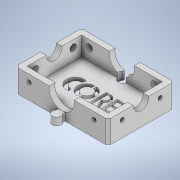
# Autodesk Inventor part: Rack holder aluminium
Saved by Autodesk Inventor 2021 (Build 250183000, 183)
## iProperties
Created: 2021-05-21
Part Number: Rack holder aluminium
Material: Generic
Document SubType Name: Modeling
Designer: Olivi
Density: 1 g/cm^3
Appearance: Default
Author: Olivi
Autodesk Inventor part; units mm, degrees
ref_plane "YZ Plane" through (0, 0, 0) normal (1, 0, 0) x (0, 1, 0)
ref_plane "XZ Plane" through (0, 0, 0) normal (0, 1, 0) x (-1, 0, 0)
ref_plane "XY Plane" through (0, 0, 0) normal (0, 0, 1) x (1, 0, 0)
sketch "Sketch1" plane through (0, 0, 0) normal (0, 1, 0) x (-1, 0, 0)
  line L0 (0, 0) -> (0, -86)
  line L1 (0, -86) -> (128.3, -86)
  line L2 (128.3, -86) -> (128.3, 0)
  line L3 (128.3, 0) -> (0, 0)
  dimension "d0" = 86
  dimension "d1" = 128.3
  constraints: 8 end point, 3 perpendicular, 1 vertical
  measures "d0" distance of L0.start L0.end
  measures "d1" distance of L0.end L1.end
extrude "Extrusion2" add sketch "Sketch1" along normal blind 6
sketch "Sketch3" plane through (0, 6, 0) normal (0, 1, 0) x (1, 0, 0)
  point P0 (0, 0)
sketch "Sketch4" plane through (0, 6, 0) normal (0, 1, 0) x (1, 0, 0)
  arc A0 (-91.2531, 56.696) -> (-91.5743, 29.7143) centre (-95.2962, 43.2514) ccw
  arc A1 (-93.1804, 51.2354) -> (-93.1804, 34.2112) centre (-94.0166, 42.7233) ccw
  line L0 (-93.1804, 51.2354) -> (-91.2531, 56.696)
  line L1 (-93.1804, 34.2112) -> (-91.5743, 29.7143)
  arc A2 (-78.0632, 52.0407) -> (-78.3199, 34.448) centre (-76.5372, 43.2202) ccw
  arc A3 (-74.7545, 34.448) -> (-75.0113, 52.0407) centre (-76.5372, 43.2202) ccw
  arc A4 (-75.0113, 29.7143) -> (-75.0113, 56.696) centre (-76.1328, 43.2051) ccw
  line L2 (-75.0113, 56.696) -> (-75.0113, 52.0407)
  line L3 (-74.7545, 34.448) -> (-75.0113, 29.7143)
  line L4 (-78.3199, 34.448) -> (-78.3199, 29.4603)
  line L5 (-78.0632, 56.6961) -> (-78.0632, 52.0407)
  arc A5 (-78.0632, 56.6961) -> (-78.3199, 29.4603) centre (-77.9302, 43.0757) ccw
  line L6 (-59.5494, 56.6961) -> (-59.5494, 29.4603)
  line L7 (-59.5494, 29.4603) -> (-55.5494, 29.4603)
  line L8 (-55.5494, 29.4603) -> (-55.5494, 56.6961)
  line L9 (-55.5494, 56.6961) -> (-59.5494, 56.6961)
  line L10 (-47.4135, 29.4603) -> (-53.7861, 43.0782)
  arc A6 (-53.7861, 43.0782) -> (-53.7861, 54.3684) centre (-53.0876, 48.7233) ccw
  line L11 (-47.4135, 29.4603) -> (-43.9803, 31.0669)
  line L12 (-43.9803, 31.0669) -> (-48.5954, 40.9288)
  arc A7 (-48.5954, 40.9288) -> (-53.7861, 56.6961) centre (-52.5494, 48.3652) ccw
  line L13 (-53.7861, 56.6961) -> (-53.7861, 54.3684)
  line L14 (-41.5494, 56.0046) -> (-41.5494, 29.4603)
  line L15 (-41.5494, 29.4603) -> (-27.5494, 29.4603)
  line L16 (-27.5494, 29.4603) -> (-27.5494, 33.1666)
  line L17 (-27.5494, 33.1666) -> (-37.5494, 33.1666)
  line L18 (-37.5494, 33.1666) -> (-37.5494, 41.4179)
  line L19 (-37.5494, 41.4179) -> (-29.2175, 41.4179)
  line L20 (-29.2175, 41.4179) -> (-29.2175, 44.4179)
  line L21 (-29.2175, 44.4179) -> (-37.5494, 44.4179)
  line L22 (-37.5494, 44.4179) -> (-37.5494, 52.4179)
  line L23 (-37.5494, 52.4179) -> (-27.5494, 52.4179)
  line L24 (-27.5494, 52.4179) -> (-27.5494, 56.0046)
  line L25 (-27.5494, 56.0046) -> (-41.5494, 56.0046)
  line L26 (-128.3, 86) -> (-128.3, 0) projected
  line L27 (0, 86) -> (-128.3, 86) projected
  point P0 (0, 0)
  constraints: 52 end point, 19 point on circle, 13 perpendicular, 8 centre point, 6 vertical, 5 point on line, 1 concentric
extrude "Extrusion3" cut sketch "Sketch4" against normal through all
sketch "Sketch26" plane through (0, 6, 0) normal (0, 1, 0) x (1, 0, 0)
  point P0 (0, 0)
sketch "Sketch27" plane through (0, 6, 0) normal (0, 1, 0) x (1, 0, 0)
  line L0 (-1.7618, -2.4025) -> (1.922, -2.4025)
  point P0 (0, 0)
  constraints: 2 end point, 1 horizontal
sketch "Sketch28" plane through (0, 6, 0) normal (0, 1, 0) x (1, 0, 0)
  point P0 (0, 0)
sketch "Sketch29" plane through (0, 6, 0) normal (0, 1, 0) x (1, 0, 0)
  line L0 (0, 86) -> (-128.3, 86) projected
  line L1 (-128.3, 86) -> (0, 86)
  line L2 (-128.3, 0) -> (0, 0) projected
  line L3 (0, 86) -> (0, 0)
  line L4 (0, 0) -> (-128.3, 0)
  line L5 (-128.3, 0) -> (-128.3, 86)
  line L6 (-137.3, -9) -> (-137.3, 95)
  line L7 (-137.3, 95) -> (9, 95)
  line L8 (9, 95) -> (9, -9)
  line L9 (9, -9) -> (-137.3, -9)
  dimension "d114" = 9
  dimension "d115" = 9
  dimension "d116" = 9
  dimension "d117" = 9
  constraints: 16 end point, 4 perpendicular, 2 collinear, 1 parallel, 1 vertical
  measures "d114" distance between parallel lines of L0 L7
  measures "d115" distance between parallel lines of L8 L3
  measures "d116" distance between parallel lines of L5 L6
  measures "d117" distance between parallel lines of L9 L2
extrude "Extrusion11" add sketch "Sketch29" along normal blind 30 and the other way blind 6
sketch "Sketch30" plane through (-137.3, 36, 9) normal (0, 0, 1) x (1, 0, 0)
  line L0 (9, 0) -> (137.3, 0) projected
  arc A0 (53.4147, 0) -> (92.5853, 0) centre (73, -4.0519) ccw
  line L1 (53.4147, 0) -> (92.5853, 0)
  line L2 (0, -36) -> (0, 0) projected
  point P0 (137.3, -36)
  dimension "d160" = 20
  dimension "d161" = 73
  constraints: 2 end point, 2 point on circle, 2 point on line, 1 centre point, 1 collinear
  measures "d160" radius of A0
  measures "d161" distance from line of A0.centre L2
extrude "Extrusion12" cut sketch "Sketch30" against normal through all
sketch "Sketch31" plane through (-137.3, 0, 9) normal (0, 0, 1) x (1, 0, 0)
  circle A0 centre (21.5643, 25) radius 3.25
  circle A1 centre (124.1286, 25) radius 3.25
  line L0 (146.3, 0) -> (0, 0) projected
  point P0 (137.3, 0)
  dimension "d124" = 6.5
  dimension "d125" = 6.5
  dimension "d126" = 25
  dimension "d127" = 25
  constraints: 2 centre point
  measures "d124" diameter of A0
  measures "d125" diameter of A1
  measures "d126" distance from line of L0 A1.centre
  measures "d127" distance from line of L0 A0.centre
extrude "Extrusion13" cut sketch "Sketch31" against normal through all
sketch "Sketch32" plane through (-128.3, 6, -86) normal (0, 0, 1) x (1, 0, 0)
  circle A0 centre (115.1286, 19) radius 3.25 projected
  circle A1 centre (115.1286, 19) radius 5.25
  circle A2 centre (12.5643, 19) radius 3.25 projected
  circle A3 centre (12.5643, 19) radius 5.25
  point P0 (128.3, -6)
  dimension "d130" = 10.5
  dimension "d131" = 10.5
  constraints: 2 centre point, 2 coincident
  measures "d130" diameter of A1
  measures "d131" diameter of A3
extrude "Extrusion14" cut sketch "Sketch32" against normal blind 6.2
sketch "Sketch33" plane through (0, 6, 0) normal (0, 0, -1) x (-1, 0, 0)
  circle A0 centre (13.1714, 19) radius 3.25 projected
  circle A1 centre (13.1714, 19) radius 5.25
  circle A2 centre (115.7357, 19) radius 3.25 projected
  circle A3 centre (115.7357, 19) radius 5.25
  point P0 (0, -6)
  dimension "d134" = 10.5
  dimension "d135" = 10.5
  constraints: 2 centre point, 2 coincident
  measures "d134" diameter of A1
  measures "d135" diameter of A3
extrude "Extrusion15" cut sketch "Sketch33" against normal blind 6.2
sketch "Sketch34" plane through (-137.3, 0, 9) normal (-1, 0, 0) x (0, 0, 1)
  line L0 (-9, 36) -> (-95, 36) projected
  line L1 (-104, 0) -> (-104, 36) projected
  arc A0 (-64.5, 36) -> (-39.5, 36) centre (-52, 34.966) ccw
  point P0 (-9, 0)
  dimension "d143" = 25
  constraints: 2 point on circle, 2 point on line, 1 centre point
  measures "d143" distance of A0.end A0.start
extrude "Extrusion16" cut sketch "Sketch34" against normal through all
sketch "Sketch35" plane through (-137.3, 0, -95) normal (-1, 0, 0) x (0, 0, 1)
  circle A0 centre (82, 25) radius 3.25
  circle A1 centre (22, 25) radius 3.25
  line L0 (104, 0) -> (0, 0) projected
  line L1 (0, 0) -> (0, 36) projected
  point P0 (95, 0)
  dimension "d144" = 6.5
  dimension "d145" = 6.5
  dimension "d146" = 25
  dimension "d147" = 25
  dimension "d150" = 60
  dimension "d151" = 22
  constraints: 2 centre point
  measures "d144" diameter of A0
  measures "d145" diameter of A1
  measures "d146" distance from line of L0 A0.centre
  measures "d147" distance from line of L0 A1.centre
  measures "d150" distance of A0.centre A1.centre
  measures "d151" distance from line of L1 A1.centre
extrude "Extrusion17" cut sketch "Sketch35" against normal through all
sketch "Sketch36" plane through (0, 6, -86) normal (-1, 0, 0) x (0, 0, 1)
  circle A0 centre (13, 19) radius 3.25 projected
  circle A1 centre (13, 19) radius 5.25
  circle A2 centre (73.1913, 19) radius 5.25
  point P0 (86, -6)
  dimension "d152" = 10.5
  dimension "d153" = 10.5
  constraints: 2 centre point, 1 coincident
  measures "d152" diameter of A1
  measures "d153" diameter of A2
extrude "Extrusion18" cut sketch "Sketch36" against normal blind 6.2 contours A0 | A1 | A2
sketch "Sketch37" plane through (-128.3, 6, 0) normal (1, 0, 0) x (0, 0, -1)
  circle A0 centre (13, 19) radius 3.25 projected
  circle A1 centre (13, 19) radius 5.25
  circle A2 centre (73, 19) radius 3.25 projected
  circle A3 centre (73, 19) radius 5.25
  point P0 (0, -6)
  dimension "d156" = 10.5
  dimension "d157" = 10.5
  constraints: 2 centre point, 2 coincident
  measures "d156" diameter of A1
  measures "d157" diameter of A3
extrude "Extrusion19" cut sketch "Sketch37" against normal blind 6.2 contours A0 | A1 | A2 | A3
sketch "Sketch39" plane through (0, 0, 0) normal (0, -1, 0) x (1, 0, 0)
  line L0 (-84.3, 9) -> (-44.3, 9) projected
  line L1 (-64.3, 9) -> (-69.3, 9)
  line L2 (-69.3, 9) -> (-69.3, 12.3114)
  line L3 (-69.3, 12.3114) -> (-59.3, 12.3114)
  line L4 (-59.3, 12.3114) -> (-59.3, 9)
  arc A0 (-59.3, 12.3114) -> (-69.3, 12.3114) centre (-64.3, 17.2104) ccw
  line L5 (-64.3, -95.7654) -> (-69.3, -95.7654)
  line L6 (-69.3, -95.7654) -> (-69.3, -92.2822)
  line L7 (-69.3, -92.2822) -> (-59.3, -92.2822)
  line L8 (-59.3, -92.2822) -> (-59.3, -95.7654)
  arc A1 (-59.3, -92.2822) -> (-69.3, -92.2822) centre (-64.3, -87.3832) ccw
  line L9 (-59.3, -95.7654) -> (-64.3, -95.7654)
  line L10 (-44.3, -95) -> (-84.3, -95) projected
  point P0 (0, 0)
  point P1 (-44.7147, 9)
  point P2 (-83.8853, 9)
  point P3 (-83.8853, -95)
  point P4 (-44.7147, -95)
  point P5 (-69.3, -95)
  point P6 (-59.3, -95)
  dimension "d162" = 5
  dimension "d163" = 10
  dimension "d164" = 7
  dimension "d165" = 5
  dimension "d166" = 10
  dimension "d167" = 7
  dimension "d168" = 0
  constraints: 18 end point, 5 perpendicular, 4 point on circle, 2 centre point, 2 point on line, 1 midpoint, 1 parallel
  measures "d162" distance of L1.start L1.end
  measures "d163" distance of L2.end L3.end
  measures "d164" radius of A0
  measures "d165" distance of L5.start L5.end
  measures "d166" distance of L6.end L7.end
  measures "d167" radius of A1
  measures "d168" horizontal distance of A0.centre A1.centre
extrude "Extrusion20" cut sketch "Sketch39" against normal blind 20 contours L6 L7 L8 L10 | A1 L7
sketch "Sketch40" plane through (0, 0, 0) normal (0, -1, 0) x (1, 0, 0)
  line L0 (-84.2, 8.8958) -> (-44.2, 8.8958)
  line L1 (-64.2, 8.8958) -> (-69.2, 8.8958)
  line L2 (-69.2, 8.8958) -> (-69.2, 12.2072)
  line L3 (-69.2, 12.2072) -> (-59.2, 12.2072)
  line L4 (-59.2, 12.2072) -> (-59.2, 8.8958)
  arc A0 (-59.2, 12.2072) -> (-69.2, 12.2072) centre (-64.2, 17.1062) ccw
  line L5 (-64.2, -95.7654) -> (-69.3, -95.7654)
  line L6 (-69.3, -95.7654) -> (-69.3, -92.2822)
  line L7 (-69.3, -92.2822) -> (-59.1, -92.2822)
  line L8 (-59.1, -92.2822) -> (-59.1, -95.7654)
  arc A1 (-59.1, -92.2822) -> (-69.3, -92.2822) centre (-64.2, -86.7831) ccw
  line L9 (-59.1, -95.7654) -> (-64.2, -95.7654)
  line L10 (-44.3, -95) -> (-84.3, -95)
  point P0 (0, 0)
  point P1 (0, 0)
  point P2 (-44.7147, 9)
  point P3 (-83.8853, 9)
  point P4 (-44.2, 8.8958)
  point P5 (-83.8853, -95)
  point P6 (-44.7147, -95)
  point P7 (-69.3, -95)
  point P8 (-59.3, -95)
  dimension "d171" = 5
  dimension "d172" = 10
  dimension "d173" = 7
  dimension "d174" = 5.1
  dimension "d175" = 10.2
  dimension "d176" = 7.5
  dimension "d177" = 0
  dimension "d187" = 10.2
  constraints: 20 end point, 4 perpendicular, 4 point on circle, 2 centre point, 1 parallel, 1 vertical, 6 other
  measures "d171" distance of L1.start L1.end
  measures "d172" distance of L2.end L3.end
  measures "d173" radius of A0
  measures "d174" distance of L5.start L5.end
  measures "d175" distance of L6.end L7.end
  measures "d176" radius of A1
  measures "d177" horizontal distance of A0.centre A1.centre
  measures "d187" distance of L8.end L5.end
extrude "Extrusion21" add sketch "Sketch40" against normal blind 12 contours L2 L3 L4 L0 | A0 L3
chamfer "Chamfer1" distance 4 angle 45 2 edges at (9, 18, 9) (9, 18, -95)
chamfer "Chamfer2" distance 4 angle 45 2 edges at (-137.3, 18, 9) (-137.3, 18, -95)
body "Solid2"
